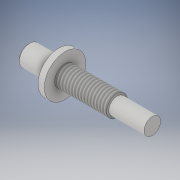
# Autodesk Inventor part: Small Gear Shaft
Saved by Autodesk Inventor 2019 (Build 230136000, 136)
## iProperties
Created: 2021-06-06
Part Number: Small Gear Shaft
Material: Generic
Document SubType Name: Modeling
Designer: micha
Density: 1 g/cm^3
Appearance: Default
Author: micha
Autodesk Inventor part; units mm, degrees
ref_plane "YZ Plane" through (0, 0, 0) normal (1, 0, 0) x (0, 1, 0)
ref_plane "XZ Plane" through (0, 0, 0) normal (0, 1, 0) x (-1, 0, 0)
ref_plane "XY Plane" through (0, 0, 0) normal (0, 0, 1) x (1, 0, 0)
sketch "Sketch1" plane through (0, 0, 0) normal (0, 0, 1) x (1, 0, 0)
  line L0 (0, 0) -> (60, 0)
  line L1 (0, 5) -> (0, 0)
  line L2 (0, 5) -> (15, 5)
  line L3 (15, 5) -> (15, 10)
  line L4 (15, 10) -> (18, 10)
  line L5 (18, 10) -> (18, 5)
  line L6 (15, 5) -> (0, 5)
  line L7 (18, 5) -> (43, 5)
  line L8 (43, 5) -> (43, 4)
  line L9 (43, 4) -> (60, 4)
  line L10 (60, 4) -> (60, 0)
  dimension "d6" = 15
  dimension "d7" = 5
  dimension "d8" = 3
  dimension "d9" = 25
  dimension "d10" = 1
  dimension "d11" = 17
  dimension "d12" = 4
  dimension "d13" = 5
  constraints: 22 end point, 5 perpendicular, 2 horizontal, 2 vertical, 1 parallel
  measures "d6" distance of L1.start L2.end
  measures "d7" distance of L2.end L3.end
  measures "d8" distance of L3.end L4.end
  measures "d9" distance of L5.end L7.end
  measures "d10" distance of L7.end L8.end
  measures "d11" distance of L8.end L9.end
  measures "d12" distance of L9.end L0.end
  measures "d13" distance between parallel lines of L7 L4
revolve "Revolution1" add sketch "Sketch1" angle 360 about axis through (0, 0, 0) along (1, 0, 0)
chamfer "Chamfer1" distance 1 angle 45 1 edges at (0, -5, 0)
thread "Thread1" size "M10x1.5" class "6g" standard "ANSI Metric M Profile" full length
body "Solid1"
